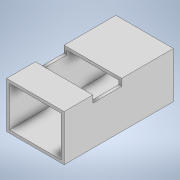
# Autodesk Inventor part: pyrodrone battery shield
Saved by Autodesk Inventor 2020 (Build 240168000, 168)
## iProperties
Created: 2021-05-15
Part Number: pyrodrone battery shield
Material: Generic
Document SubType Name: Modeling
Designer: Steven
Density: 1 g/cm^3
Appearance: Default
Author: Steven
Autodesk Inventor part; units mm, degrees
ref_plane "YZ Plane" through (0, 0, 0) normal (1, 0, 0) x (0, 1, 0)
ref_plane "XZ Plane" through (0, 0, 0) normal (0, 1, 0) x (-1, 0, 0)
ref_plane "XY Plane" through (0, 0, 0) normal (0, 0, 1) x (1, 0, 0)
sketch "Sketch1" plane through (0, 0, 0) normal (0, 1, 0) x (-1, 0, 0)
  line L0 (0, 0) -> (-50, 0)
  line L1 (-50, 0) -> (-50, -95)
  line L2 (-50, -95) -> (0, -95)
  line L3 (0, -95) -> (0, 0)
  dimension "d0" = 50
  dimension "d1" = 95
  constraints: 8 end point, 3 perpendicular, 1 horizontal
  measures "d0" distance of L0.start L0.end
  measures "d1" distance of L0.end L1.end
extrude "Extrusion1" add sketch "Sketch1" along normal blind 40
sketch "Sketch2" plane through (0, 0, 0) normal (0, 0, 1) x (1, 0, 0)
  line L0 (0, 0) -> (50, 0) construction
  line L1 (50, 0) -> (50, 40) construction
  line L2 (0, 40) -> (50, 40) construction
  line L3 (0, 0) -> (0, 40) construction
  line L4 (47.5, 37.5) -> (47.5, 2.5)
  line L5 (47.5, 2.5) -> (2.5, 2.5)
  line L6 (2.5, 2.5) -> (2.5, 37.5)
  line L7 (2.5, 37.5) -> (47.5, 37.5)
  dimension "d4" = 2.5
  dimension "d5" = 45
  dimension "d6" = 35
  constraints: 8 end point, 3 other
  measures "d4" distance between parallel lines of L2 L7
  measures "d5" distance of L6.end L4.start
  measures "d6" distance of L4.start L4.end
extrude "Extrusion2" cut sketch "Sketch2" against normal blind 90
sketch "Sketch3" plane through (0, 40, 0) normal (0, 1, 0) x (1, 0, 0)
  line L0 (50, 0) -> (50, 95) construction
  line L1 (50, 95) -> (0, 95) construction
  line L2 (0, 95) -> (0, 0) construction
  line L3 (0, 0) -> (50, 0) construction
  line L4 (50, 95) -> (0, 95) construction
  line L5 (25, 95) -> (25, 50) construction
  line L6 (25, 95) -> (25, 25) construction
  line L7 (25, 50) -> (50, 50)
  line L8 (50, 50) -> (50, 25)
  line L9 (50, 0) -> (50, 95) projected
  line L10 (50, 25) -> (0, 25)
  line L11 (0, 25) -> (0, 50)
  line L12 (0, 95) -> (0, 0) projected
  line L13 (0, 50) -> (25, 50)
  dimension "d9" = 45
  dimension "d10" = 70
  constraints: 14 end point, 5 point on line, 3 perpendicular, 2 vertical, 1 midpoint
  measures "d9" distance of L5.start L5.end
  measures "d10" distance of L5.start L6.end
extrude "Extrusion3" cut sketch "Sketch3" against normal blind 6
sketch "Sketch4" plane through (50, 0, -95) normal (0, 0, -1) x (-1, 0, 0)
  line L0 (0, 0) -> (50, 0) construction
  line L1 (50, 0) -> (50, 40) construction
  line L2 (0, 40) -> (50, 40) construction
  line L3 (0, 0) -> (0, 40) construction
  line L4 (0, 40) -> (50, 40) construction
  line L5 (25, 40) -> (25, 0) construction
  line L6 (50, 0) -> (0, 0) construction
  circle A0 centre (25, 20) radius 12.5
  dimension "d13" = 25
  constraints: 3 midpoint, 2 end point, 1 centre point
  measures "d13" diameter of A0
extrude "Extrusion4" cut sketch "Sketch4" against normal up to next
body "Solid1"
